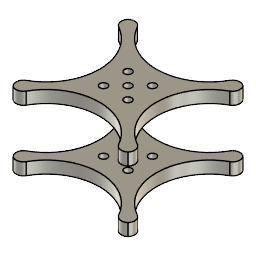
can v10 (Autodesk Fusion 360 archive; units mm, degrees)
design "vib iso"
Autodesk Fusion 360 part; units mm, degrees
sketch "Sketch1" plane through (0, 0, 0) normal (0, 0, 1) x (1, 0, 0)
  line L0 (0, 0) -> (1.5, 0)
  line L1 (0, 1.5) -> (0, 0)
  line L2 (0, 0) -> (-1.5, 0)
  line L3 (0, 1.5) -> (0, 0)
  line L4 (0, 0) -> (-1.5, 0)
  line L5 (0, -1.5) -> (0, 0)
  line L6 (0, 0) -> (1.5, 0)
  line L7 (0, -1.5) -> (0, 0)
  arc A0 (18.9092, -22.7557) -> (0, -11.6667) centre (0, -33.3333) ccw
  arc A1 (11.6667, 0) -> (22.7557, -18.9092) centre (33.3333, 0) ccw
  arc A2 (18.9092, -22.7557) -> (23.8185, -23.2278) centre (21.5274, -21.2911) ccw
  arc A3 (23.2278, -23.8185) -> (22.7557, -18.9092) centre (21.2911, -21.5274) ccw
  arc A4 (11.6667, 0) -> (22.7557, -18.9092) centre (33.3333, 0) ccw
  arc A5 (18.9092, -22.7557) -> (0, -11.6667) centre (0, -33.3333) ccw
  arc A6 (18.9092, -22.7557) -> (23.8185, -23.2278) centre (21.5274, -21.2911) ccw
  arc A7 (23.2278, -23.8185) -> (22.7557, -18.9092) centre (21.2911, -21.5274) ccw
  arc A8 (18.9092, -22.7557) -> (0, -11.6667) centre (0, -33.3333) ccw
  arc A9 (18.9092, -22.7557) -> (0, -11.6667) centre (0, -33.3333) ccw
  arc A10 (11.6667, 0) -> (22.7557, -18.9092) centre (33.3333, 0) ccw
  arc A11 (18.9092, 22.7557) -> (0, 11.6667) centre (0, 33.3333) cw
  arc A12 (18.9092, 22.7557) -> (0, 11.6667) centre (0, 33.3333) cw
  arc A13 (11.6667, 0) -> (22.7557, 18.9092) centre (33.3333, 0) cw
  arc A14 (23.2278, 23.8185) -> (22.7557, 18.9092) centre (21.2911, 21.5274) cw
  arc A15 (18.9092, 22.7557) -> (23.8185, 23.2278) centre (21.5274, 21.2911) cw
  arc A16 (-18.9092, 22.7557) -> (0, 11.6667) centre (0, 33.3333) ccw
  arc A17 (-18.9092, 22.7557) -> (-23.8185, 23.2278) centre (-21.5274, 21.2911) ccw
  arc A18 (-23.2278, 23.8185) -> (-22.7557, 18.9092) centre (-21.2911, 21.5274) ccw
  arc A19 (-11.6667, 0) -> (-22.7557, 18.9092) centre (-33.3333, 0) ccw
  arc A20 (-11.6667, 0) -> (-22.7557, -18.9092) centre (-33.3333, 0) cw
  arc A21 (-18.9092, -22.7557) -> (0, -11.6667) centre (0, -33.3333) cw
  arc A22 (-23.2278, -23.8185) -> (-22.7557, -18.9092) centre (-21.2911, -21.5274) cw
  arc A23 (-18.9092, -22.7557) -> (-23.8185, -23.2278) centre (-21.5274, -21.2911) cw
  circle A24 centre (-5, 5) radius 1.5
  circle A25 centre (5, 5) radius 1.5
  circle A26 centre (-5, -5) radius 1.5
  circle A27 centre (5, -5) radius 1.5
  circle A28 centre (0, 0) radius 1.5
  dimension "d2" = 3
  dimension "d4" = 3
  dimension "d5" = 3
  dimension "d6" = 3
  dimension "d7" = 3
  dimension "d8" = 3
  dimension "d9" = 3
  dimension "d10" = 3
  dimension "d11" = 3
  dimension "d12" = 3
  constraint coincident L0.start L1.end
  constraint tangent A0 A2
  constraint tangent A1 A3
  constraint equal A2 A3
  constraint tangent A5 A6
  constraint tangent A4 A7
  constraint equal A6 A7
  constraint coincident A28 L1.start
  constraint coincident A28 L0.end
  constraint coincident A28 L5.start
  constraint coincident A28 L2.end
  measures "d2" radius of A2
  measures "d4" radius of A6
  measures "d5" radius of A15
  measures "d6" radius of A23
  measures "d7" radius of A17
  measures "d8" diameter of A24
  measures "d9" diameter of A25
  measures "d10" diameter of A26
  measures "d11" diameter of A27
  measures "d12" diameter of A28
extrude "Extrude1" add sketch "Sketch1" along normal blind 5 makes body 1
copy_body "CopyPasteBodies1" bodies 1 makes body 2
move_body "Move1" bodies 2 to x (1, 0, 0) y (0, 1, 0) z (0, 0, 1) at (0, 0, 25)
